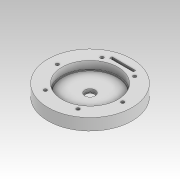
# Autodesk Inventor part: Wrist_planetary
Saved by Autodesk Inventor 2020 (Build 240168000, 168)
## iProperties
Created: 2021-03-19
Part Number: Wrist_planetary
Material: Generic
Document SubType Name: Modeling
Designer: DDeGo
Density: 1 g/cm^3
Appearance: Default
Author: DDeGo
Autodesk Inventor part; units mm, degrees
ref_plane "YZ Plane" through (0, 0, 0) normal (1, 0, 0) x (0, 1, 0)
ref_plane "XZ Plane" through (0, 0, 0) normal (0, 1, 0) x (-1, 0, 0)
ref_plane "XY Plane" through (0, 0, 0) normal (0, 0, 1) x (1, 0, 0)
sketch "Sketch19" plane through (0, 0, 0) normal (1, 0, 0) x (0, 1, 0)
  line L0 (0, 0) -> (14.81, 0) construction
  line L1 (0, 0) -> (0, 4.6) construction
  line L2 (0, 29.5) -> (1, 29.5)
  line L3 (1, 29.5) -> (1, 40.5)
  line L4 (1, 40.5) -> (0, 40.5)
  line L5 (0, 40.5) -> (0, 45)
  line L6 (0, 45) -> (12.5, 45)
  line L7 (12.5, 45) -> (12.5, 30)
  line L8 (12.5, 30) -> (4.5, 30)
  line L9 (4.5, 30) -> (4.5, 29)
  line L10 (4.5, 29) -> (3.5, 29)
  line L11 (3.5, 29) -> (3.5, 5.6)
  line L12 (3.5, 5.6) -> (0.5, 5.6)
  line L13 (0.5, 5.6) -> (0.5, 4.6)
  line L14 (0.5, 4.6) -> (0, 4.6)
  line L15 (0, 4.6) -> (0, 29.5)
  dimension "d90" = 0.5
  dimension "d91" = 5.6
  dimension "d92" = 1
  dimension "d93" = 29.5
  dimension "d94" = 40.5
  dimension "d95" = 45
  dimension "d96" = 1
  dimension "d97" = 1
  dimension "d99" = 30
  dimension "d100" = 1
  dimension "d101" = 8
  dimension "d103" = 3
  constraints: 32 end point, 14 perpendicular, 2 point on line, 2 vertical, 1 horizontal
  measures "d90" distance of L13.end L1.end
  measures "d91" distance between parallel lines of L0 L12
  measures "d92" distance of L12.end L13.end
  measures "d93" distance between parallel lines of L0 L2
  measures "d94" distance between parallel lines of L0 L4
  measures "d95" distance between parallel lines of L0 L6
  measures "d96" distance of L9.end L10.end
  measures "d97" distance of L8.end L9.end
  measures "d99" distance between parallel lines of L0 L8
  measures "d100" distance between parallel lines of L15 L3
  measures "d101" distance of L7.end L8.end
  measures "d103" distance between parallel lines of L11 L13
revolve "Revolution2" add sketch "Sketch19" angle 360 about axis through (0, 0, 0) along (0, 1, 0)
sketch "Sketch20" plane through (0, 12.5, 0) normal (0, 1, 0) x (1, 0, 0)
  circle A0 centre (0, 0) radius 35 construction
  circle A1 centre (35, 0) radius 1.75
  dimension "d104" = 70
  dimension "d105" = 3.5
  constraints: 2 horizontal alignment, 1 centre point, 1 coincident, 2 other
  measures "d105" diameter of A1
extrude "Extrusion18" cut sketch "Sketch20" against normal through all
sketch "Sketch21" plane through (0, 1, 0) normal (0, -1, 0) x (1, 0, 0)
  line L0 (32.1, 2.9) -> (37.9, 2.9)
  line L1 (37.9, 2.9) -> (37.9, -2.9)
  line L2 (37.9, -2.9) -> (32.1, -2.9)
  line L3 (32.1, -2.9) -> (32.1, 2.9)
  circle A0 centre (35, 0) radius 1.75 projected
  line L4 (32.1, 2.9) -> (37.9, -2.9) construction
  line L5 (37.9, 2.9) -> (32.1, -2.9) construction
  point P0 (0, 0)
  dimension "d108" = 5.8
  dimension "d109" = 5.8
  constraints: 12 end point, 2 midpoint, 2 parallel, 1 horizontal, 1 perpendicular
  measures "d108" distance of L1.end L2.end
  measures "d109" distance of L0.end L1.end
extrude "Extrusion19" cut sketch "Sketch21" against normal blind 3 contours L0 L1 L2 L3 | A0
pattern_circular "Circular Pattern3" count 6 over 360 about axis through (0, 6.25, 0) along (0, 1, 0) of "Extrusion19", "Extrusion18"
sketch "Sketch22" plane through (0, 12.5, 0) normal (0, 1, 0) x (1, 0, 0)
  line L0 (-12.7, 36.27) -> (12.7, 36.27)
  line L1 (12.7, 36.27) -> (12.7, 33.73)
  line L2 (12.7, 33.73) -> (-12.7, 33.73)
  line L3 (-12.7, 33.73) -> (-12.7, 36.27)
  line L4 (-12.7, 36.27) -> (12.7, 33.73) construction
  line L5 (12.7, 36.27) -> (-12.7, 33.73) construction
  line L6 (0, 35) -> (0, 0) construction
  dimension "d115" = 35
  dimension "d116" = 25.4
  dimension "d117" = 2.54
  constraints: 14 end point, 2 midpoint, 2 parallel, 2 perpendicular, 1 horizontal
  measures "d115" distance of L6.end L6.start
  measures "d116" distance of L0.start L0.end
  measures "d117" distance of L0.end L1.end
extrude "Extrusion20" cut sketch "Sketch22" against normal through all
body "Solid2"
